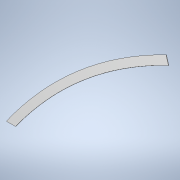
# Autodesk Inventor part: thirdseatbeltpart
Saved by Autodesk Inventor 2021 (Build 250183000, 183)
## iProperties
Created: 2020-10-12
Part Number: thirdseatbeltpart
Material: Generic
Document SubType Name: Modeling
Designer: atwaterh
Density: 1 g/cm^3
Appearance: Default
Author: atwaterh
Autodesk Inventor part; units mm, degrees
ref_plane "YZ Plane" through (0, 0, 0) normal (1, 0, 0) x (0, 1, 0)
ref_plane "XZ Plane" through (0, 0, 0) normal (0, 1, 0) x (-1, 0, 0)
ref_plane "XY Plane" through (0, 0, 0) normal (0, 0, 1) x (1, 0, 0)
sketch "Sketch1" plane through (0, 0, 0) normal (0, 1, 0) x (-1, 0, 0)
  line L0 (0, 0) -> (50.8, 0)
  line L1 (50.8, 0) -> (50.8, -2.54)
  line L2 (50.8, -2.54) -> (0, -2.54)
  line L3 (0, -2.54) -> (0, 0)
  dimension "d0" = 50.8
  dimension "d1" = 2.54
  constraints: 8 end point, 3 perpendicular, 1 horizontal
  measures "d0" distance of L0.start L0.end
  measures "d1" distance of L0.end L1.end
sketch3d "3D Sketch1"
  spline S0 degree 2 poles (0, 0, 0) (75.4249, 208.3087, -262.555) (339.4126, 209.5254, -506.007) knots 1 1 1 2 2 2
sweep "Sweep1" add profiles "Sketch1" path "3D Sketch1"
body "Solid1"
